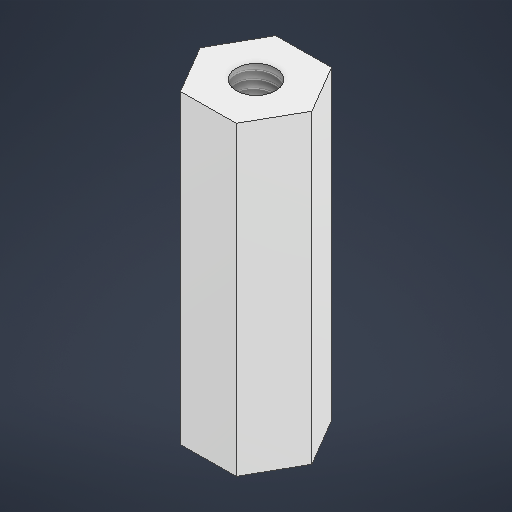
# Autodesk Inventor part: pataUnion
Saved by Autodesk Inventor 2026.1 (Build 301233020, 233B)
## iProperties
Created: 2025-10-27
Part Number: pataUnion
Material: Poliestireno
Document SubType Name: Modeling
Designer: rodri
Density: 1.021 g/cm^3
Appearance: Suave - Blanco
Author: rodri
Autodesk Inventor part; units mm, degrees
ref_plane "YZ Plane" through (0, 0, 0) normal (1, 0, 0) x (0, 1, 0)
ref_plane "XZ Plane" through (0, 0, 0) normal (0, 1, 0) x (-1, 0, 0)
ref_plane "XY Plane" through (0, 0, 0) normal (0, 0, 1) x (1, 0, 0)
sketch "Boceto1" plane through (0, 0, 0) normal (0, 1, 0) x (-1, 0, 0)
  line L0 (1.7076, 3.014) -> (3.464, 0.0282)
  line L1 (3.464, 0.0282) -> (1.7564, -2.9858)
  line L2 (1.7564, -2.9858) -> (-1.7076, -3.014)
  line L3 (-1.7076, -3.014) -> (-3.464, -0.0282)
  line L4 (-3.464, -0.0282) -> (-1.7564, 2.9858)
  line L5 (-1.7564, 2.9858) -> (1.7076, 3.014)
  point P0 (0, 0)
  point P1 (0, 0)
  dimension "d0" = 6
  constraints: 12 end point, 1 coincident, 13 other
  measures "d0" distance between parallel lines of L3 L0
extrude "Extrusión1" add sketch "Boceto1" along normal blind 19.1
sketch "Boceto2" plane through (0, 19.1, 0) normal (0, 1, 0) x (1, 0, 0)
  point P0 (0, 0)
  point P1 (0, 0)
  constraints: 1 coincident
hole "Agujero1" at (0, 19.1, 0) direction (0, -1, 0) diameter 2.459 end through all thread size "M3x0.5" class "6H" standard "ISO Metric profile"
